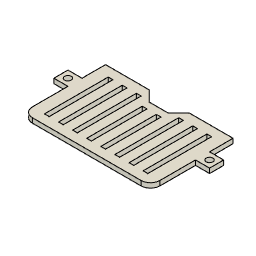
Stepper_Hood_v10 (Autodesk Fusion 360 design; units mm, degrees)
Autodesk Fusion 360 part; units mm, degrees
sketch "Sketch1" plane through (0, 0, 0) normal (0, 1, 0) x (1, 0, 0)
  line L0 (0, 12.575) -> (27.15, 12.575) construction
  line L1 (27.15, 12.575) -> (27.15, -8.575)
  line L2 (23.15, -12.575) -> (0, -12.575)
  line L3 (27.15, 12.575) -> (33.15, 12.575)
  line L4 (33.15, 12.575) -> (33.15, 6.575)
  line L5 (33.15, 6.575) -> (27.15, 6.575)
  line L6 (27.15, 6.575) -> (27.15, 12.575)
  line L7 (0, -12.575) -> (0, 12.575) construction
  circle A0 centre (30.15, 9.575) radius 1.425
  line L8 (27.15, 6.575) -> (33.15, 12.575) construction
  arc A1 (23.15, -12.575) -> (27.15, -8.575) centre (23.15, -8.575) ccw
  line L9 (-27.15, 12.575) -> (-27.15, -8.575)
  line L10 (-33.15, 6.575) -> (-27.15, 6.575)
  circle A2 centre (-30.15, 9.575) radius 1.425
  line L11 (-27.15, 12.575) -> (-33.15, 12.575)
  line L12 (-33.15, 12.575) -> (-33.15, 6.575)
  line L13 (-23.15, -12.575) -> (0, -12.575)
  arc A3 (-27.15, -8.575) -> (-23.15, -12.575) centre (-23.15, -8.575) ccw
  line L14 (-27.15, 0) -> (27.15, 0) construction
  line L15 (-27.15, 12.575) -> (-27.15, 22.575)
  line L16 (-27.15, 22.575) -> (27.15, 22.575)
  line L17 (27.15, 22.575) -> (27.15, 12.575)
  line L18 (-10, -8.575) -> (-10, 18.575)
  line L19 (-10, 18.575) -> (-8, 18.575)
  line L20 (-8, 18.575) -> (-8, -8.575)
  line L21 (-8, -8.575) -> (-10, -8.575)
  line L22 (-16, -8.575) -> (-16, 18.575)
  line L23 (-16, 18.575) -> (-14, 18.575)
  line L24 (-14, 18.575) -> (-14, -8.575)
  line L25 (-14, -8.575) -> (-16, -8.575)
  line L26 (-22, -8.575) -> (-22, 18.575)
  line L27 (-22, 18.575) -> (-20, 18.575)
  line L28 (-20, 18.575) -> (-20, -8.575)
  line L29 (-20, -8.575) -> (-22, -8.575)
  line L30 (-4, 18.075) -> (4, 18.075)
  line L31 (-4, 18.075) -> (-8.5, 22.575)
  line L32 (4, 18.075) -> (8.5, 22.575)
  line L33 (20, -8.575) -> (22, -8.575)
  line L34 (14, -8.575) -> (16, -8.575)
  line L35 (8, 18.575) -> (8, -8.575)
  line L36 (22, 18.575) -> (20, 18.575)
  line L37 (10, 18.575) -> (8, 18.575)
  line L38 (8, -8.575) -> (10, -8.575)
  line L39 (16, -8.575) -> (16, 18.575)
  line L40 (22, -8.575) -> (22, 18.575)
  line L41 (14, 18.575) -> (14, -8.575)
  line L42 (16, 18.575) -> (14, 18.575)
  line L43 (10, -8.575) -> (10, 18.575)
  line L44 (20, 18.575) -> (20, -8.575)
  line L45 (-4, 15.075) -> (-2, 15.075)
  line L46 (-2, 15.075) -> (-2, -8.575)
  line L47 (-2, -8.575) -> (-4, -8.575)
  line L48 (-4, -8.575) -> (-4, 15.075)
  line L49 (4, 15.075) -> (2, 15.075)
  line L50 (2, 15.075) -> (2, -8.575)
  line L51 (4, -8.575) -> (4, 15.075)
  line L52 (2, -8.575) -> (4, -8.575)
  point P0 (23.15, -8.575)
  point P1 (0, 18.075)
  dimension "d1" = 6
  dimension "d2" = 6
  dimension "d4" = 33.15
  dimension "d5" = 2.85
  dimension "d6" = 4
  dimension "d16" = 10
  dimension "d18" = 25.15
  dimension "d25" = 4.5
  dimension "d26" = 45
  dimension "d27" = 45
  dimension "d28" = 2
  dimension "d29" = 8
  dimension "d30" = 27.15
  dimension "d31" = 4
  dimension "d32" = 4
  dimension "d33" = 4
  dimension "d34" = 8
  dimension "d35" = 4
  dimension "d36" = 3
  constraint horizontal L0
  constraint vertical L1
  constraint horizontal L2
  constraint horizontal L3
  constraint vertical L4
  constraint horizontal L5
  constraint vertical L6
  constraint coincident L1 L0.end
  constraint perpendicular L0 L7
  constraint midpoint origin L7
  constraint collinear L0 L3
  constraint midpoint A0.centre L8
  constraint tangent L1 A1
  constraint tangent L2 A1
  constraint symmetric L0.end L7 L9.start
  constraint symmetric L2.end L7 L13.end
  constraint symmetric L3.end L7 L11.end
  constraint symmetric L4.end L7 L10.start
  constraint symmetric L5.end L7 L10.end
  constraint symmetric L7 A0 A2
  constraint symmetric L7 L1.end L9.end
  constraint symmetric L7 L2.start L13.start
  constraint symmetric L7 A1 A3
  constraint coincident L9 L14.start
  constraint coincident L1 L14.end
  constraint perpendicular L1 L14
  constraint midpoint origin L14
  constraint perpendicular L11 L15
  constraint perpendicular L15 L16
  constraint vertical L17
  constraint coincident L16 L31.end
  constraint coincident L16 L32.end
  constraint perpendicular L19 L20
  constraint perpendicular L18 L21
  constraint perpendicular L18 L19
  constraint equal L21 L25
  constraint equal L25 L29
  constraint equal L18 L22
  constraint equal L22 L26
  constraint equal L24 L28
  constraint equal L20 L24
  constraint horizontal L25
  constraint horizontal L29
  constraint horizontal L22.start L28.end
  constraint horizontal L18.start L24.end
  constraint perpendicular L22 L23
  constraint perpendicular L27 L28
  constraint perpendicular L26 L27
  constraint vertical L24
  constraint symmetric L7 A3.centre P0
  constraint symmetric L7 L18.start L38.end
  constraint symmetric L7 L18.end L37.start
  constraint symmetric L7 L19.end L35.start
  constraint symmetric L7 L20.end L35.end
  constraint symmetric L7 L22.start L34.end
  constraint symmetric L7 L22.end L39.end
  constraint symmetric L7 L23.end L41.start
  constraint symmetric L7 L24.end L34.start
  constraint symmetric L7 L26.start L33.end
  constraint symmetric L7 L26.end L36.start
  constraint symmetric L7 L27.end L36.end
  constraint symmetric L7 L28.end L33.start
  constraint midpoint L30 P1
  constraint vertical origin P1
  constraint horizontal L45
  constraint vertical L46
  constraint horizontal L47
  constraint vertical L48
  constraint equal L21 L47
  constraint horizontal L20.end L47.end
  constraint symmetric L7 L45.start L49.start
  constraint symmetric L7 L45.end L49.end
  constraint symmetric L7 L46.end L50.end
  constraint symmetric L7 L47.end L51.start
  measures "d1" distance of L3.end L4.end
  measures "d2" distance of L4 L6
  measures "d4" distance of origin L4
  measures "d5" diameter of A0
  measures "d6" radius of A1
  measures "d16" distance of L9.start L15.end
  measures "d18" distance of L0.start L2.end
  measures "d25" distance of L16 L30
  measures "d26" angle of L16 L31
  measures "d27" angle of L16 L32
  measures "d28" distance of L18.start L20.end
  measures "d29" distance of origin L20
  measures "d30" distance of L18.start L18.end
  measures "d31" distance of L13 L21
  measures "d32" distance of L18 L24
  measures "d33" distance of L22 L28
  measures "d34" distance of L30.start L30.end
  measures "d35" distance of L20 L48
  measures "d36" distance of L30 L45
extrude "Extrude1" add sketch "Sketch1" along normal blind 2 contours L1 L3 L4 L5 L6 | L1 L2 L6 A1 L9 L13 A3 L15 L16 L17 L30 L31 L32 | L9 L10 L11 L12
